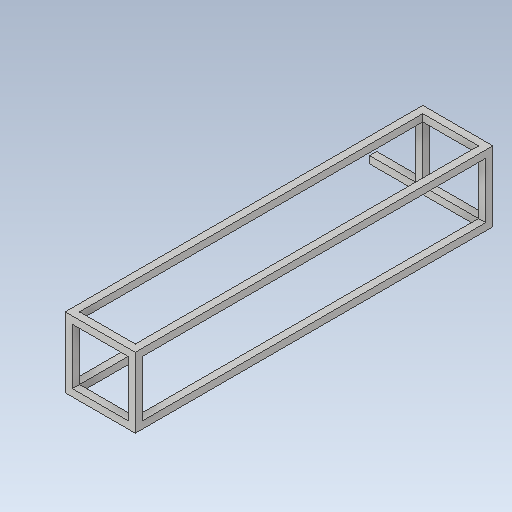
# Autodesk Inventor part: Accumalator Housing
Saved by Autodesk Inventor 2020 (Build 240168000, 168)
## iProperties
Created: 2020-10-15
Part Number: Accumalator Housing
Material: Generic
Document SubType Name: Modeling
Designer: nabee
Density: 1 g/cm^3
Appearance: Default
Author: nabee
Autodesk Inventor part; units mm, degrees
ref_plane "YZ Plane" through (0, 0, 0) normal (1, 0, 0) x (0, 1, 0)
ref_plane "XZ Plane" through (0, 0, 0) normal (0, 1, 0) x (-1, 0, 0)
ref_plane "XY Plane" through (0, 0, 0) normal (0, 0, 1) x (1, 0, 0)
sketch "Sketch1" plane through (0, 0, 0) normal (0, 0, 1) x (1, 0, 0)
  line L0 (0, 0) -> (68, 0)
  line L1 (68, 0) -> (68, 68)
  line L2 (68, 68) -> (0, 68)
  line L3 (0, 68) -> (0, 0)
  dimension "d1" = 68
  dimension "d2" = 68
  constraints: 8 end point, 2 parallel, 1 horizontal, 1 perpendicular
  measures "d1" distance of L0.start L0.end
  measures "d2" distance of L2.end L0.start
extrude "Extrusion1" add sketch "Sketch1" along normal blind 480
sketch "Sketch2" plane through (0, 0, 480) normal (0, 0, 1) x (1, 0, 0)
  line L0 (10, 58) -> (58, 58)
  line L1 (58, 58) -> (58, 10)
  line L2 (58, 10) -> (10, 10)
  line L3 (10, 10) -> (10, 58)
  line L4 (68, 68) -> (0, 68) projected
  line L5 (0, 68) -> (0, 0) projected
  line L6 (0, 0) -> (68, 0) projected
  line L7 (68, 0) -> (68, 68) projected
  dimension "d5" = 10
  dimension "d6" = 10
  dimension "d7" = 10
  dimension "d8" = 10
  constraints: 8 end point, 2 parallel, 1 horizontal, 1 perpendicular
  measures "d5" distance between parallel lines of L4 L0
  measures "d6" distance between parallel lines of L5 L3
  measures "d7" distance between parallel lines of L6 L2
  measures "d8" distance between parallel lines of L7 L1
extrude "Extrusion2" cut sketch "Sketch2" against normal blind 900 contours L0 L1 L2 L3
sketch "Sketch3" plane through (68, 0, 0) normal (1, 0, 0) x (0, 0, -1)
  line L0 (-470, 58) -> (-10, 58)
  line L1 (-10, 58) -> (-10, 10)
  line L2 (-10, 10) -> (-470, 10)
  line L3 (-470, 10) -> (-470, 58)
  line L4 (0, 68) -> (-480, 68) projected
  line L5 (-480, 0) -> (-480, 68) projected
  line L6 (0, 0) -> (-480, 0) projected
  line L7 (0, 0) -> (0, 68) projected
  dimension "d11" = 10
  dimension "d12" = 10
  dimension "d13" = 10
  dimension "d14" = 10
  constraints: 8 end point, 2 parallel, 1 horizontal, 1 perpendicular
  measures "d11" distance between parallel lines of L4 L0
  measures "d12" distance between parallel lines of L5 L3
  measures "d13" distance between parallel lines of L6 L2
  measures "d14" distance between parallel lines of L7 L1
extrude "Extrusion3" cut sketch "Sketch3" against normal blind 900 contours L0 L1 L2 L3
sketch "Sketch4" plane through (0, 68, 0) normal (0, 1, 0) x (1, 0, 0)
  line L0 (68, -10) -> (58, -10) projected
  line L1 (10, -480) -> (10, -470) projected
  line L2 (58, -10) -> (10, -10)
  line L3 (10, -10) -> (10, -470)
  line L4 (10, -470) -> (58, -470)
  line L5 (58, -470) -> (58, -10)
  point P0 (0, 0)
  constraints: 8 end point, 2 parallel, 1 horizontal, 1 perpendicular
extrude "Extrusion4" cut sketch "Sketch4" against normal blind 900
sketch "Sketch5" plane through (0, 0, 480) normal (0, 0, 1) x (1, 0, 0)
  line L0 (68, 68) -> (0, 68) projected
  line L1 (0, 0) -> (68, 0) projected
  line L2 (0, 68) -> (68, 68)
  line L3 (68, 68) -> (68, 0)
  line L4 (68, 0) -> (0, 0)
  line L5 (0, 0) -> (0, 68)
  line L6 (10, 58) -> (0, 58) projected
  line L7 (58, 58) -> (58, 10) projected
  line L8 (10, 58) -> (58, 58)
  line L9 (58, 58) -> (58, 10)
  line L10 (58, 10) -> (10, 10)
  line L11 (10, 10) -> (10, 58)
  constraints: 16 end point, 4 parallel, 2 horizontal, 2 perpendicular
extrude "Extrusion5" add sketch "Sketch5" along normal blind 10
sketch "Sketch6" plane through (0, 68, 0) normal (0, 1, 0) x (1, 0, 0)
  line L0 (58, -490) -> (58, -470) projected
  line L1 (10, -490) -> (10, -470) projected
  line L2 (58, -470) -> (10, -470)
  line L3 (10, -470) -> (10, -480)
  line L4 (10, -480) -> (58, -480)
  line L5 (58, -480) -> (58, -470)
  point P0 (0, 0)
  constraints: 8 end point, 2 parallel, 1 horizontal, 1 midpoint, 1 perpendicular
extrude "Extrusion6" cut sketch "Sketch6" against normal blind 900
sketch "Sketch7" plane through (68, 0, 0) normal (1, 0, 0) x (0, 0, -1)
  line L0 (-470, 10) -> (-470, 58) projected
  line L1 (-480, 10) -> (-480, 0) projected
  line L2 (-470, 58) -> (-480, 58)
  line L3 (-480, 58) -> (-480, 10)
  line L4 (-480, 10) -> (-470, 10)
  line L5 (-470, 10) -> (-470, 58)
  point P0 (0, 0)
  constraints: 8 end point, 2 parallel, 1 horizontal, 1 perpendicular
extrude "Extrusion7" cut sketch "Sketch7" against normal blind 900
sketch "Sketch8" plane through (0, 0, 0) normal (0, 0, -1) x (-1, 0, 0)
  line L0 (-68, 0) -> (-68, 68) projected
  line L1 (-68, 68) -> (0, 68)
  line L2 (0, 68) -> (0, 0)
  line L3 (0, 0) -> (-68, 0)
  line L4 (-68, 0) -> (-68, 68)
  line L5 (-58, 58) -> (-10, 58)
  line L6 (-10, 58) -> (-10, 10)
  line L7 (-10, 10) -> (-58, 10)
  line L8 (-58, 10) -> (-58, 58)
  constraints: 16 end point, 4 parallel, 2 horizontal, 2 perpendicular
extrude "Extrusion8" add sketch "Sketch8" along normal blind 10
sketch "Sketch9" plane through (0, 68, 490) normal (0, 1, 0) x (1, 0, 0)
  line L0 (10, 480) -> (10, 500) projected
  line L1 (58, 480) -> (58, 500) projected
  line L2 (10, 480) -> (58, 480)
  line L3 (58, 480) -> (58, 490)
  line L4 (58, 490) -> (10, 490)
  line L5 (10, 490) -> (10, 480)
  point P0 (0, 490)
  constraints: 8 end point, 2 parallel, 1 horizontal, 1 midpoint, 1 perpendicular
extrude "Extrusion9" cut sketch "Sketch9" against normal blind 900
sketch "Sketch10" plane through (68, 0, 490) normal (1, 0, 0) x (0, 0, -1)
  line L0 (10, 58) -> (480, 58) projected
  line L1 (490, 10) -> (500, 10) projected
  line L2 (480, 58) -> (490, 58)
  line L3 (490, 58) -> (490, 10)
  line L4 (490, 10) -> (480, 10)
  line L5 (480, 10) -> (480, 58)
  point P0 (490, 0)
  constraints: 8 end point, 2 parallel, 1 horizontal, 1 perpendicular
extrude "Extrusion10" cut sketch "Sketch10" against normal blind 900
sketch "Sketch11" plane through (68, 0, 490) normal (1, 0, 0) x (0, 0, -1)
  line L0 (0, 68) -> (0, 0) projected
  line L1 (500, 0) -> (500, 68) projected
  line L2 (0, 68) -> (500, 68)
  line L3 (500, 68) -> (500, 0)
  line L4 (500, 0) -> (0, 0)
  line L5 (0, 0) -> (0, 68)
  line L6 (490, 58) -> (490, 10) projected
  line L7 (10, 58) -> (490, 58)
  line L8 (490, 58) -> (490, 10)
  line L9 (490, 10) -> (10, 10)
  line L10 (10, 10) -> (10, 58)
  point P0 (490, 0)
  constraints: 16 end point, 4 parallel, 2 horizontal, 2 perpendicular
extrude "Extrusion11" add sketch "Sketch11" along normal blind 20
sketch "Sketch12" plane through (0, 68, 490) normal (0, 1, 0) x (1, 0, 0)
  line L0 (58, 10) -> (58, 490) projected
  line L1 (88, 490) -> (58, 490) projected
  line L2 (58, 10) -> (78, 10)
  line L3 (78, 10) -> (78, 490)
  line L4 (78, 490) -> (58, 490)
  line L5 (58, 490) -> (58, 10)
  point P0 (0, 490)
  dimension "d33" = 20
  constraints: 8 end point, 2 parallel, 1 horizontal, 1 perpendicular, 1 point on line
  measures "d33" distance of L4.end L3.end
extrude "Extrusion12" cut sketch "Sketch12" against normal blind 900
sketch "Sketch13" plane through (0, 0, -10) normal (0, 0, -1) x (-1, 0, 0)
  line L0 (-58, 58) -> (-10, 58) projected
  line L1 (-58, 58) -> (-78, 58)
  line L2 (-78, 58) -> (-78, 10)
  line L3 (-78, 10) -> (-58, 10)
  line L4 (-58, 10) -> (-58, 58)
  point P0 (0, 0)
  dimension "d36" = 20
  constraints: 8 end point, 2 parallel, 1 horizontal, 1 perpendicular
  measures "d36" distance of L3.end L2.end
extrude "Extrusion13" cut sketch "Sketch13" against normal blind 900
sketch "Sketch14" plane through (0, 68, 490) normal (0, 1, 0) x (1, 0, 0)
  line L0 (0, 0) -> (88, 0) projected
  line L1 (0, 500) -> (88, 500) projected
  line L2 (0, 0) -> (88, 0)
  line L3 (88, 0) -> (88, 500)
  line L4 (88, 500) -> (0, 500)
  line L5 (0, 500) -> (0, 0)
  line L6 (10, 10) -> (10, 490) projected
  line L7 (78, 10) -> (78, 490) projected
  line L8 (10, 10) -> (78, 10)
  line L9 (78, 10) -> (78, 490)
  line L10 (78, 490) -> (10, 490)
  line L11 (10, 490) -> (10, 10)
  point P0 (0, 490)
  constraints: 16 end point, 4 parallel, 2 horizontal, 2 perpendicular
extrude "Extrusion14" add sketch "Sketch14" along normal blind 10
sketch "Sketch15" plane through (88, 0, 490) normal (1, 0, 0) x (0, 0, -1)
  line L0 (10, 58) -> (490, 58) projected
  line L1 (490, 78) -> (490, 58) projected
  line L2 (10, 58) -> (490, 58)
  line L3 (490, 58) -> (490, 68)
  line L4 (490, 68) -> (10, 68)
  line L5 (10, 68) -> (10, 58)
  point P0 (490, 0)
  constraints: 8 end point, 2 parallel, 1 horizontal, 1 midpoint, 1 perpendicular
extrude "Extrusion15" cut sketch "Sketch15" against normal blind 900
sketch "Sketch16" plane through (0, 0, -10) normal (0, 0, -1) x (-1, 0, 0)
  line L0 (-78, 10) -> (-78, 58) projected
  line L1 (-10, 68) -> (0, 68) projected
  line L2 (-78, 58) -> (-10, 58)
  line L3 (-10, 58) -> (-10, 68)
  line L4 (-10, 68) -> (-78, 68)
  line L5 (-78, 68) -> (-78, 58)
  point P0 (0, 0)
  constraints: 8 end point, 2 parallel, 1 horizontal, 1 perpendicular
extrude "Extrusion16" cut sketch "Sketch16" against normal blind 900
sketch "Sketch17" plane through (0, 78, 490) normal (0, 1, 0) x (1, 0, 0)
  line L0 (88, 0) -> (88, 500) projected
  line L1 (0, 0) -> (88, 0) projected
  line L2 (88, 500) -> (0, 500)
  line L3 (0, 500) -> (0, 0)
  line L4 (0, 0) -> (88, 0)
  line L5 (88, 0) -> (88, 500)
  line L6 (78, 490) -> (78, 10) projected
  line L7 (10, 10) -> (10, 490) projected
  line L8 (78, 490) -> (10, 490)
  line L9 (10, 490) -> (10, 10)
  line L10 (10, 10) -> (78, 10)
  line L11 (78, 10) -> (78, 490)
  point P0 (0, 490)
  constraints: 16 end point, 4 parallel, 2 horizontal, 2 perpendicular
extrude "Extrusion17" add sketch "Sketch17" along normal blind 20
sketch "Sketch18" plane through (88, 0, 490) normal (1, 0, 0) x (0, 0, -1)
  line L0 (490, 68) -> (10, 68) projected
  line L1 (10, 68) -> (490, 68)
  line L2 (490, 68) -> (490, 88)
  line L3 (490, 88) -> (10, 88)
  line L4 (10, 88) -> (10, 68)
  point P0 (490, 0)
  dimension "d47" = 20
  constraints: 8 end point, 2 parallel, 1 horizontal, 1 perpendicular
  measures "d47" distance of L1.end L2.end
extrude "Extrusion18" cut sketch "Sketch18" against normal blind 900
sketch "Sketch19" plane through (0, 0, 490) normal (0, 0, 1) x (1, 0, 0)
  line L0 (10, 68) -> (10, 10) projected
  line L1 (78, 88) -> (78, 98) projected
  line L2 (10, 68) -> (78, 68)
  line L3 (78, 68) -> (78, 88)
  line L4 (78, 88) -> (10, 88)
  line L5 (10, 88) -> (10, 68)
  point P0 (0, 0)
  constraints: 8 end point, 2 parallel, 1 horizontal, 1 perpendicular
extrude "Extrusion19" cut sketch "Sketch19" against normal blind 900
sketch "Sketch20" plane through (0, 0, -10) normal (-1, 0, 0) x (0, 0, 1)
  line L0 (0, 98) -> (500, 98) projected
  line L1 (0, 98) -> (500, 98)
  line L2 (500, 98) -> (500, 0)
  line L3 (500, 0) -> (0, 0)
  line L4 (0, 0) -> (0, 98)
  line L5 (10, 88) -> (490, 88) projected
  line L6 (490, 10) -> (10, 10) projected
  line L7 (10, 88) -> (490, 88)
  line L8 (490, 88) -> (490, 10)
  line L9 (490, 10) -> (10, 10)
  line L10 (10, 10) -> (10, 88)
  point P0 (10, 0)
  constraints: 16 end point, 4 parallel, 2 horizontal, 2 perpendicular
extrude "Extrusion20" add sketch "Sketch20" along normal blind 10
sketch "Sketch21" plane through (0, 0, 490) normal (0, 0, 1) x (1, 0, 0)
  line L0 (78, 88) -> (10, 88) projected
  line L1 (10, 10) -> (-10, 10) projected
  line L2 (10, 88) -> (0, 88)
  line L3 (0, 88) -> (0, 10)
  line L4 (0, 10) -> (10, 10)
  line L5 (10, 10) -> (10, 88)
  point P0 (0, 0)
  constraints: 8 end point, 2 parallel, 1 horizontal, 1 midpoint, 1 perpendicular
extrude "Extrusion21" cut sketch "Sketch21" against normal blind 900
sketch "Sketch22" plane through (0, 98, 490) normal (0, 1, 0) x (1, 0, 0)
  line L0 (10, 490) -> (78, 490) projected
  line L1 (0, 10) -> (-10, 10) projected
  line L2 (10, 490) -> (0, 490)
  line L3 (0, 490) -> (0, 10)
  line L4 (0, 10) -> (10, 10)
  line L5 (10, 10) -> (10, 490)
  point P0 (0, 490)
  constraints: 8 end point, 2 parallel, 1 horizontal, 1 perpendicular
extrude "Extrusion22" cut sketch "Sketch22" against normal blind 900
sketch "Sketch24" plane through (-10, 0, -10) normal (-1, 0, 0) x (0, 0, 1)
  line L0 (500, 0) -> (0, 0) projected
  line L1 (10, 88) -> (10, 10) projected
  line L2 (0, 0) -> (10, 0)
  line L3 (10, 0) -> (10, 10)
  line L4 (10, 10) -> (0, 10)
  line L5 (0, 10) -> (0, 0)
  point P0 (10, 0)
  constraints: 8 end point, 2 parallel, 1 horizontal, 1 perpendicular
extrude "Extrusion24" add sketch "Sketch24" along normal blind 64.455
body "Solid1"
